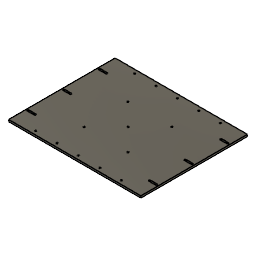
RampenPlatte (Autodesk Fusion 360 design; units mm, degrees)
Autodesk Fusion 360 part; units mm, degrees
sketch "Skizze1" plane through (0, 0, 0) normal (0, 0, 1) x (1, 0, 0)
  line L0 (0, 0) -> (278, 0)
  line L1 (278, 0) -> (278, 224)
  line L2 (278, 224) -> (0, 224)
  line L3 (0, 224) -> (0, 0)
  line L4 (0, 112) -> (4, 112) construction
  line L5 (139, 224) -> (139, 0) construction
  line L6 (4, 110.35) -> (19, 110.35)
  arc A0 (19, 110.35) -> (19, 113.65) centre (19, 112) ccw
  line L7 (19, 113.65) -> (4, 113.65)
  arc A1 (4, 113.65) -> (4, 110.35) centre (4, 112) ccw
  line L8 (4, 112) -> (19, 112) construction
  line L9 (0, 187) -> (4, 187) construction
  line L10 (4, 185.35) -> (19, 185.35)
  arc A2 (19, 185.35) -> (19, 188.65) centre (19, 187) ccw
  line L11 (19, 188.65) -> (4, 188.65)
  arc A3 (4, 188.65) -> (4, 185.35) centre (4, 187) ccw
  line L12 (4, 187) -> (19, 187) construction
  line L13 (19, 35.35) -> (4, 35.35)
  arc A4 (4, 38.65) -> (4, 35.35) centre (4, 37) ccw
  arc A5 (19, 35.35) -> (19, 38.65) centre (19, 37) ccw
  line L14 (4, 38.65) -> (19, 38.65)
  line L15 (4, 37) -> (19, 37) construction
  line L16 (0, 37) -> (4, 37) construction
  line L17 (259, 188.65) -> (274, 188.65)
  arc A6 (274, 185.35) -> (274, 188.65) centre (274, 187) ccw
  arc A7 (259, 188.65) -> (259, 185.35) centre (259, 187) ccw
  line L18 (274, 185.35) -> (259, 185.35)
  line L19 (259, 113.65) -> (274, 113.65)
  arc A8 (274, 110.35) -> (274, 113.65) centre (274, 112) ccw
  arc A9 (259, 113.65) -> (259, 110.35) centre (259, 112) ccw
  line L20 (274, 110.35) -> (259, 110.35)
  arc A10 (259, 38.65) -> (259, 35.35) centre (259, 37) ccw
  line L21 (259, 35.35) -> (274, 35.35)
  arc A11 (274, 35.35) -> (274, 38.65) centre (274, 37) ccw
  line L22 (274, 38.65) -> (259, 38.65)
  circle A12 centre (139, 8) radius 1.65
  line L23 (139, 112) -> (200, 112) construction
  circle A13 centre (49, 8) radius 1.65
  circle A14 centre (94, 8) radius 1.65
  circle A15 centre (184, 8) radius 1.65
  circle A16 centre (229, 8) radius 1.65
  circle A17 centre (139, 216) radius 1.65
  circle A18 centre (229, 216) radius 1.65
  circle A19 centre (184, 216) radius 1.65
  circle A20 centre (49, 216) radius 1.65
  circle A21 centre (94, 216) radius 1.65
  circle A22 centre (139, 112) radius 1.65
  line L24 (139, 112) -> (184.9619, 66.0381) construction
  circle A23 centre (184.9619, 66.0381) radius 1.65
  circle A24 centre (184.9619, 157.9619) radius 1.65
  line L25 (139, 112) -> (184.9619, 157.9619) construction
  circle A25 centre (93.0381, 157.9619) radius 1.65
  line L26 (139, 112) -> (93.0381, 157.9619) construction
  circle A26 centre (93.0381, 66.0381) radius 1.65
  line L27 (139, 112) -> (93.0381, 66.0381) construction
  dimension "d1" = 224
  dimension "d2" = 278
  dimension "d3" = 3.3
  dimension "d4" = 15
  dimension "d5" = 4
  dimension "d6" = 150
  dimension "d9" = 3.3
  dimension "d10" = 8
  dimension "d13" = 90
  dimension "d14" = 0
  dimension "d15" = 3.3
  dimension "d19" = 45
  dimension "d20" = 3.3
  dimension "d22" = 360
  dimension "d23" = 130
  constraint horizontal L0
  constraint vertical L1
  constraint horizontal L2
  constraint vertical L3
  constraint coincident L0.start L3.end
  constraint midpoint L3 L4.start
  constraint perpendicular L3 L4
  constraint midpoint L2 L5.start
  constraint midpoint L0 L5.end
  constraint tangent L6 A0
  constraint tangent A0 L7
  constraint parallel L6 L7
  constraint tangent L7 A1
  constraint tangent L6 A1
  constraint perpendicular L3 L8
  constraint coincident L4.end A1.centre
  constraint coincident L3 L9.start
  constraint perpendicular L3 L9
  constraint tangent L10 A2
  constraint tangent A2 L11
  constraint parallel L10 L11
  constraint tangent L11 A3
  constraint tangent L10 A3
  constraint perpendicular L3 L12
  constraint coincident L9.end A3.centre
  constraint equal A0 A2
  constraint equal L6 L10
  constraint equal L4 L9
  constraint symmetric L8 L9.start L16.start
  constraint symmetric L8 L9.end A4.centre
  constraint symmetric L8 L10.start A4.start
  constraint symmetric L8 L10.end A5.end
  constraint symmetric L8 A2.end L13.start
  constraint symmetric L8 L11.end L13.end
  constraint symmetric L8 A2 A5
  constraint symmetric L8 A3 A4
  constraint symmetric L5 L6.start A8.start
  constraint symmetric L5 L6.end A9.end
  constraint symmetric L5 A0.end L19.start
  constraint symmetric L5 L7.end L19.end
  constraint symmetric L5 A0 A9
  constraint symmetric L5 A1 A8
  constraint symmetric L5 L10.start A6.start
  constraint symmetric L5 L10.end A7.end
  constraint symmetric L5 A2.end L17.start
  constraint symmetric L5 L11.end L17.end
  constraint symmetric L5 A2 A7
  constraint symmetric L5 A3 A6
  constraint symmetric L5 L13.start A10.end
  constraint symmetric L5 L13.end L21.end
  constraint symmetric L5 A4.start A11.end
  constraint symmetric L5 A4 A11
  constraint symmetric L5 A5.end A10.start
  constraint symmetric L5 A5 A10
  constraint coincident L5 A12.centre
  constraint midpoint L5 L23.start
  constraint perpendicular L5 L23
  constraint symmetric A12 L23 A17
  constraint symmetric L23 A13 A20
  constraint symmetric L23 A14 A21
  constraint symmetric L23 A15 A19
  constraint symmetric L23 A16 A18
  constraint coincident L23.start A22.centre
  constraint coincident L24.end A23.centre
  measures "d1" distance of L0.start L2.end
  measures "d2" distance of L0.start L0.end
  measures "d3" distance of L6 L7
  measures "d4" distance of L4.end A0.centre
  measures "d5" distance of L4.start L4.end
  measures "d6" distance of L12 L15
  measures "d9" diameter of A12
  measures "d10" distance of L0 A12.centre
  measures "d15" diameter of A22
  measures "d19" angle of L23 L24
  measures "d20" diameter of A23
  measures "d23" distance of L24.end A25.centre
extrude "Extrusion1" add sketch "Skizze1" along normal blind 4
